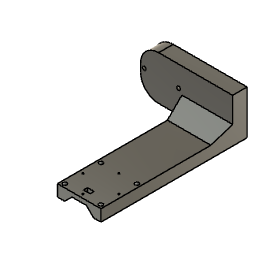
Pan Tilt Large Drone Mount v11 (Autodesk Fusion 360 design; units mm, degrees)
Autodesk Fusion 360 part; units mm, degrees
sketch "Sketch1" plane through (0, 0, 0) normal (0, 1, 0) x (1, 0, 0)
  line L0 (0, 0) -> (67.945, 0)
  line L1 (67.945, 0) -> (67.945, -10.16)
  line L2 (67.945, -10.16) -> (0, -10.16)
  line L3 (0, -10.16) -> (0, 0)
  line L4 (0, -10.16) -> (10.16, -10.16)
  line L5 (10.16, -10.16) -> (10.16, 0)
  line L6 (10.16, 0) -> (0, 0)
  line L7 (0, 0) -> (0, -10.16)
  line L8 (67.945, -10.16) -> (57.785, -10.16)
  line L9 (57.785, -10.16) -> (57.785, 0)
  line L10 (57.785, 0) -> (67.945, 0)
  line L11 (67.945, 0) -> (67.945, -10.16)
  point P0 (3.81, -5.08)
  point P1 (64.135, -5.08)
  dimension "d1" = 60.325
  dimension "d2" = 5.08
  dimension "d3" = 5.08
  dimension "d4" = 3.81
  dimension "d5" = 3.81
  constraint horizontal P0 P1
  constraint horizontal L0
  constraint vertical L1
  constraint horizontal L2
  constraint vertical L3
  constraint coincident L0.start L3.end
  constraint horizontal L4
  constraint vertical L5
  constraint horizontal L6
  constraint vertical L7
  constraint horizontal L8
  constraint vertical L9
  constraint horizontal L10
  constraint vertical L11
  constraint collinear L0 L10
  constraint collinear L0 L6
  constraint equal L8 L9
  constraint equal L5 L6
  measures "d1" distance of P0 P1
  measures "d2" distance of P1 L0
  measures "d3" distance of P1 L2
  measures "d4" distance of P1 L1
  measures "d5" distance of P0 L3
extrude "Extrude1" add sketch "Sketch1" along normal blind 6.35 contours L0 L2 L3 L4 L5 L6 L7 | L0 L1 L2 L8 L9 L10 L11 makes body 1 at (3.3867, 0, 3.3867) makes body 2 at (64.5583, 0, 3.3867)
extrude "Extrude2" add sketch "Sketch1" against normal blind 2.286 bodies 1 2
sketch "Sketch2" plane through (0, -2.286, 0) normal (0, -1, 0) x (1, 0, 0)
  line L0 (67.945, 0) -> (67.945, 10.16)
  line L1 (0, 10.16) -> (0, 0)
  line L2 (158.75, -35.56) -> (158.75, -15.24)
  line L3 (158.75, -15.24) -> (82.55, -15.24)
  line L4 (82.55, -15.24) -> (82.55, -35.56)
  line L5 (146.05, -35.56) -> (146.05, -22.86)
  line L6 (146.05, -22.86) -> (95.25, -22.86)
  line L7 (95.25, -22.86) -> (95.25, -35.56)
  line L8 (82.55, -35.56) -> (95.25, -35.56)
  line L9 (146.05, -35.56) -> (158.75, -35.56)
  line L10 (120.65, -15.24) -> (120.65, -22.86)
  line L11 (67.945, 10.16) -> (0, 10.16)
  line L12 (82.55, -15.24) -> (158.75, -15.24)
  line L13 (158.75, -15.24) -> (158.75, 10.16)
  line L14 (158.75, 10.16) -> (82.55, 10.16)
  line L15 (82.55, 10.16) -> (82.55, -15.24)
  point P0 (33.9725, 10.16)
  point P1 (120.65, 10.16)
  dimension "d20" = 25.4
  dimension "d21" = 12.7
  dimension "d28" = 76.2
  dimension "d29" = 86.6775
  dimension "d45" = 20.32
  dimension "d103" = 7.62
  constraint horizontal L8
  constraint vertical L2
  constraint horizontal L3
  constraint vertical L4
  constraint vertical L5
  constraint horizontal L6
  constraint vertical L7
  constraint collinear L8 L9
  constraint equal L8 L9
  constraint midpoint L3 L10.start
  constraint midpoint L6 L10.end
  constraint horizontal L12
  constraint vertical L13
  constraint horizontal L14
  constraint vertical L15
  constraint coincident L11 L13.end
  constraint collinear L2 L13
  constraint midpoint L11 P0
  constraint midpoint L14 P1
  measures "d20" distance of L3 L11
  measures "d21" distance of L2.start L5.start
  measures "d28" distance of L3.end L2.end
  measures "d29" distance of P0 P1
  measures "d45" distance of L2.start L2.end
  measures "d103" distance of L10.start L10.end
extrude "Extrude3" add sketch "Sketch2" along normal blind 6.35 contours L3 L12 L13 L14 L15 bodies 1 makes body 3
extrude "Extrude4" add sketch "Sketch2" along normal blind 247.65 contours L2 L3 L5 L6 L9 L10 L12 | L3 L4 L6 L7 L8 L10 L12 bodies 3
extrude "Extrude5" add 1 faces at (67.945, 0.5927, 6.7733) along direction (1, 0, 0) blind 26.7208 on bodies 1 bodies 1 3
extrude "Extrude6" add 1 faces at (27.5167, -2.286, 3.3867) along direction (0, -1, 0) blind 6.35 on bodies 1 bodies 1
extrude "Extrude10" add 1 faces at (94.6658, 0.5927, 6.7733) along direction (1, 0, 0) blind 64.0842 on bodies 1 bodies 1
extrude "Extrude11" add 1 faces at (112.1833, -2.286, -7.62) along direction (0, 1, 0) blind 8.636 on bodies 1 bodies 1
extrude "Extrude12" add 1 faces at (125.095, -0.762, 10.16) along direction (0, 0, 1) blind 2.54 on bodies 1 bodies 1
extrude "Extrude13" add 1 faces at (74.295, -0.762, 0) along direction (0, 0, -1) blind 2.54 on bodies 1 bodies 1
extrude "Extrude14" add 1 faces at (0, 1.3547, 2.54) along direction (-1, 0, 0) blind 2.54 on bodies 1 bodies 1
sketch "Sketch5" plane through (0, 0, -15.24) normal (0, 0, 1) x (-1, 0, 0)
  line L0 (-82.55, 8.636) -> (-82.55, 249.936)
  line L1 (-82.55, 249.936) -> (-158.75, 249.936)
  line L2 (-158.75, 249.936) -> (-158.75, 8.636)
  line L3 (-89.0778, 180.2638) -> (-152.2222, 180.2638)
  line L4 (-152.2222, 180.2638) -> (-152.2222, 243.4082)
  line L5 (-152.2222, 243.4082) -> (-89.0778, 243.4082)
  line L6 (-89.0778, 243.4082) -> (-89.0778, 180.2638)
  line L7 (-89.0778, 211.836) -> (-82.55, 211.836)
  line L8 (-152.2222, 211.836) -> (-158.75, 211.836)
  line L9 (-120.65, 243.4082) -> (-120.65, 249.936)
  circle A0 centre (-120.65, 180.2638) radius 3.4925
  circle A1 centre (-120.65, 180.2638) radius 1.55
  circle A2 centre (-152.2222, 180.2638) radius 3.4925
  circle A3 centre (-152.2222, 180.2638) radius 1.55
  circle A4 centre (-152.2222, 211.836) radius 3.4925
  circle A5 centre (-152.2222, 211.836) radius 1.55
  circle A6 centre (-152.2222, 243.4082) radius 3.4925
  circle A7 centre (-152.2222, 243.4082) radius 1.55
  circle A8 centre (-120.65, 243.4082) radius 3.4925
  circle A9 centre (-120.65, 243.4082) radius 1.55
  circle A10 centre (-89.0778, 243.4082) radius 3.4925
  circle A11 centre (-89.0778, 243.4082) radius 1.55
  circle A12 centre (-89.0778, 211.836) radius 3.4925
  circle A13 centre (-89.0778, 211.836) radius 1.55
  circle A14 centre (-89.0778, 180.2638) radius 3.4925
  circle A15 centre (-89.0778, 180.2638) radius 1.55
  line L10 (-158.75, 8.636) -> (-82.55, 8.636)
  line L11 (-114.935, 229.6922) -> (-126.365, 229.6922)
  line L12 (-126.365, 229.6922) -> (-126.365, 236.5502)
  line L13 (-126.365, 236.5502) -> (-114.935, 236.5502)
  line L14 (-114.935, 236.5502) -> (-114.935, 229.6922)
  line L15 (-120.65, 236.5502) -> (-120.65, 239.9157)
  line L16 (-120.65, 239.9157) -> (-123.19, 239.9157)
  dimension "d69" = 63.1444
  dimension "d70" = 3.1
  dimension "d71" = 6.985
  dimension "d83" = 6.858
  dimension "d84" = 11.43
  dimension "d86" = 6.858
  constraint horizontal L3
  constraint vertical L4
  constraint horizontal L5
  constraint vertical L6
  constraint equal L3 L6
  constraint midpoint L6 L7.start
  constraint coincident L0 L7.end
  constraint perpendicular L0 L7
  constraint midpoint L4 L8.start
  constraint coincident L2 L8.end
  constraint perpendicular L2 L8
  constraint midpoint L5 L9.start
  constraint midpoint L1 L9.end
  constraint equal L7 L9
  constraint equal L8 L9
  constraint midpoint L3 A0.centre
  constraint concentric A0 A1
  constraint coincident L3.end L4.start
  constraint concentric A2 A3
  constraint coincident L8.start A4.centre
  constraint concentric A4 A5
  constraint coincident L4.end L5.start
  constraint concentric A6 A7
  constraint coincident L9.start A8.centre
  constraint concentric A8 A9
  constraint coincident L5.end L6.start
  constraint coincident L7.start A12.centre
  constraint concentric A12 A13
  constraint coincident L3.start L6.end
  constraint concentric A14 A15
  constraint equal A1 A15
  constraint equal A1 A3
  constraint equal A3 A5
  constraint equal A5 A7
  constraint equal A7 A9
  constraint equal A9 A11
  constraint equal A11 A13
  constraint equal A0 A14
  constraint equal A0 A2
  constraint equal A2 A4
  constraint equal A4 A6
  constraint equal A6 A8
  constraint equal A8 A10
  constraint equal A10 A12
  constraint horizontal L11
  constraint vertical L12
  constraint horizontal L13
  constraint vertical L14
  constraint midpoint L13 L15.start
  constraint coincident A8 L15.end
  constraint perpendicular L13 L15
  constraint perpendicular L15 L16
  constraint tangent A8 L16
  measures "d69" distance of L3.start L3.end
  measures "d70" diameter of A15
  measures "d71" diameter of A14
  measures "d83" distance of L11 L13
  measures "d84" distance of L12.end L13.end
  measures "d86" distance of L5 L13
extrude "Extrude16" cut sketch "Sketch5" against normal through all contours L6 L7 A13 | L6 L7 A13 | L6 A13 | L4 L8 A5 | L4 L8 A5 | L5 L9 A9 | L5 L9 A9 | L5 L6 A11 | L5 L6 A11 | L3 L6 A15 | L3 L6 A15 | L4 A5 | L5 A9 | L4 L5 A7 | L4 L5 A7 | L3 L4 A3 | L3 L4 A3 | L3 A1 | L3 A1 bodies 1
extrude "Extrude17" cut sketch "Sketch5" against normal through all from surface at -11.43 contours L6 L7 A12 A13 | L6 L7 A12 A13 | L6 A12 A13 | L4 L8 A4 A5 | L4 L8 A4 A5 | L5 L6 A10 A11 | L5 L6 A10 A11 | L3 L6 A14 A15 | L3 L6 A14 A15 | L4 A4 A5 | L4 L5 A6 A7 | L4 L5 A6 A7 | L3 L4 A2 A3 | L3 L4 A2 A3 bodies 1
extrude "Extrude18" cut sketch "Sketch5" against normal through all contours L5 L6 A10 A11 | L5 L6 A10 A11 | L3 L6 A14 A15 | L3 L6 A14 A15 | L4 L5 A6 A7 | L4 L5 A6 A7 | L3 L4 A2 A3 | L3 L4 A2 A3 bodies 1
extrude "Extrude19" cut sketch "Sketch5" against normal through all contours L11 L12 L13 L14 bodies 1
hole "Hole3" at (64.135, 0, 5.08) direction (0, -1, 0) diameter 6.35 end through all bodies 1
extrude "Extrude20" cut 1 faces at (63.3685, 0, 3.682) along direction (0, 1, 0) blind 1.27 on bodies 1 bodies 1
chamfer "Chamfer9" distance 6.35 distance2 5.08 1 edges at (10.16, 0, 5.08) measured on face at (10.16, 2.1167, 7.62) on bodies 1
chamfer "Chamfer10" distance 5.08 distance2 6.35 1 edges at (57.785, 0, 5.08) measured on face at (29.421, 0, 2.54) on bodies 1
chamfer "Chamfer11" distance 12.7 distance2 12.7 2 edges at (95.25, -121.793, -22.86) (146.05, -121.793, -22.86) measured on face at (95.25, -164.5073, -27.0933) measured on face at (120.6927, -55.3397, -22.86) on bodies 1
ref_plane "WorkPlane2" through (78.105, -1.143, 5.08) normal (0, 0, 1) x (1, 0, 0)
sketch "Sketch6" plane through (0, 0, 5.08) normal (0, 0, 1) x (1, 0, 0)
  line L0 (-2.54, -8.636) -> (70.485, -8.636)
  line L1 (70.485, -8.636) -> (70.485, 6.35)
  line L2 (70.485, 6.35) -> (-2.54, 6.35)
  line L3 (-2.54, 6.35) -> (-2.54, -8.636)
  line L4 (33.9725, 6.35) -> (33.9725, -8.636)
  line L5 (15.24, 0) -> (33.9725, 0)
  line L6 (10.16, 6.35) -> (15.24, 0)
  line L7 (10.16, 6.35) -> (15.24, 0)
  point P0 (70.485, 6.35)
  point P1 (57.785, 6.35)
  point P2 (-2.54, -8.636)
  point P3 (-2.54, -8.636)
  dimension "d95" = 12.7
  constraint horizontal P0 P1
  constraint coincident P2 L0.start
  constraint horizontal L0
  constraint vertical L1
  constraint horizontal L2
  constraint vertical L3
  constraint coincident P0 L1.end
  constraint midpoint L2 L4.start
  constraint midpoint L0 L4.end
  constraint coincident L4 L5.end
  constraint perpendicular L4 L5
  constraint coincident L2 L6.start
  constraint coincident L5.start L6.end
  constraint equal L6 L7
  measures "d95" distance of P0 P1
revolve "Revolve1" add sketch "Sketch6" angle 360 about axis through (33.9725, 6.35, 5.08) along (0, -1, 0) contours L0 L2 L3 L4 L5 L6 L7 bodies 1
hole "Hole2" at (3.81, 0, 5.08) at (64.135, 0, 5.08) direction (0, 1, 0) diameter 3.4925 end through all bodies 1
hole "Hole4" at (3.81, 0, 5.08) at (64.135, 0, 5.08) direction (0, -1, 0) diameter 6.35 end through all bodies 1
extrude "Extrude21" cut 1 faces at (64.2927, 0, 7.7669) along direction (0, 1, 0) blind 1.016 on bodies 1 bodies 1
extrude "Extrude22" add 1 faces at (33.1017, -8.636, 17.6906) along direction (0, -1, 0) blind 10.414 on bodies 1 bodies 1
sketch "Sketch7" plane through (82.55, 0, 0) normal (-1, 0, 0) x (0, -1, 0)
  line L0 (19.05, -2.54) -> (-6.35, -2.54)
  line L1 (-6.35, -2.54) -> (-6.35, -35.56)
  line L2 (-6.35, -35.56) -> (249.936, -35.56)
  line L3 (249.936, -35.56) -> (249.936, -15.24)
  line L4 (249.936, -15.24) -> (19.05, -15.24)
  line L5 (19.05, -15.24) -> (19.05, -2.54)
  line L6 (-6.35, -35.56) -> (19.05, -35.56)
  line L7 (19.05, -35.56) -> (19.05, -15.24)
  line L8 (19.05, -15.24) -> (-6.35, -15.24)
  line L9 (-6.35, -15.24) -> (-6.35, -35.56)
  constraint horizontal L6
  constraint vertical L7
  constraint horizontal L8
  constraint vertical L9
  constraint coincident L4.end L5.start
  constraint coincident L1.end L2.start
extrude "Extrude23" add sketch "Sketch7" along normal blind 24.4348 contours L0 L1 L5 L8 | L1 L2 L6 L7 L8 L9 bodies 1
sketch "Sketch8" plane through (0, 6.35, 0) normal (0, 1, 0) x (-1, 0, 0)
  circle A0 centre (-3.81, 5.08) radius 1.7463
  circle A1 centre (-64.135, 5.08) radius 1.7463
  circle A2 centre (-33.9725, 5.08) radius 23.8125
  line L0 (2.54, -2.54) -> (2.54, 12.7)
  line L1 (2.54, 12.7) -> (1.736, 12.7)
  arc A3 (1.736, 12.7) -> (-69.681, 12.7) centre (-33.9725, 5.08) ccw
  line L2 (-69.681, 12.7) -> (-158.75, 12.7)
  line L3 (-158.75, 12.7) -> (-158.75, -35.56)
  line L4 (-158.75, -35.56) -> (-146.05, -35.56)
  line L5 (-146.05, -35.56) -> (-133.35, -22.86)
  line L6 (-133.35, -22.86) -> (-107.95, -22.86)
  line L7 (-107.95, -22.86) -> (-95.25, -35.56)
  line L8 (-95.25, -35.56) -> (-58.1152, -35.56)
  line L9 (-33.9725, 41.5925) -> (-158.75, 41.5925)
  line L10 (-158.75, 41.5925) -> (-158.75, 12.7)
  line L11 (-158.75, 12.7) -> (-33.9725, 12.7)
  line L12 (-33.9725, 12.7) -> (-33.9725, 41.5925)
  line L13 (-33.9725, 41.5925) -> (2.54, 41.5925)
  line L14 (2.54, 41.5925) -> (2.54, 12.7)
  line L15 (2.54, 12.7) -> (-33.9725, 12.7)
  line L16 (-33.9725, 12.7) -> (-33.9725, 41.5925)
  line L17 (-58.1152, -35.56) -> (-58.1152, -22.3115)
  arc A4 (-58.1152, -22.3115) -> (1.736, -2.54) centre (-33.9725, 5.08) ccw
  line L18 (1.736, -2.54) -> (2.54, -2.54)
  line L19 (-58.1152, -35.56) -> (2.54, -35.56)
  line L20 (2.54, -35.56) -> (2.54, 12.7)
  line L21 (2.54, 12.7) -> (-58.1152, 12.7)
  line L22 (-58.1152, 12.7) -> (-58.1152, -35.56)
  constraint horizontal L9
  constraint vertical L10
  constraint horizontal L11
  constraint vertical L12
  constraint coincident L2.end L3.start
  constraint midpoint A3 L9.start
  constraint horizontal L13
  constraint vertical L14
  constraint horizontal L15
  constraint vertical L16
  constraint coincident L0.end L1.start
  constraint horizontal L19
  constraint vertical L20
  constraint horizontal L21
  constraint vertical L22
  constraint coincident L8.end L17.start
extrude "Extrude26" add sketch "Sketch8" against normal up to surface (25.4 mm away) contours L1 A3 L13 L14 L15 L21 | A3 L2 L9 L10 L11 | L17 A4 L18 L19 L20 L22 bodies 1
chamfer "Chamfer12" distance 38.1 distance2 12.7 2 edges at (120.65, -19.05, -15.24) (82.55, -19.05, -25.4) measured on face at (120.6114, -72.2727, -15.24) measured on face at (82.55, -96.012, -22.0133) on bodies 1
fillet "Fillet1" radius 31.75 2 edges at (-2.54, -6.35, 41.5925) (-2.54, -6.35, -35.56) on bodies 1
equation "d12 = -0.25 in + 0.16 in"
equation "d29 = ( 6.825 / 2 ) * 1 in"
equation "d69 = 2.746 in - 0.26 in"
equation "d99 = 1 in - 0.59 in"
